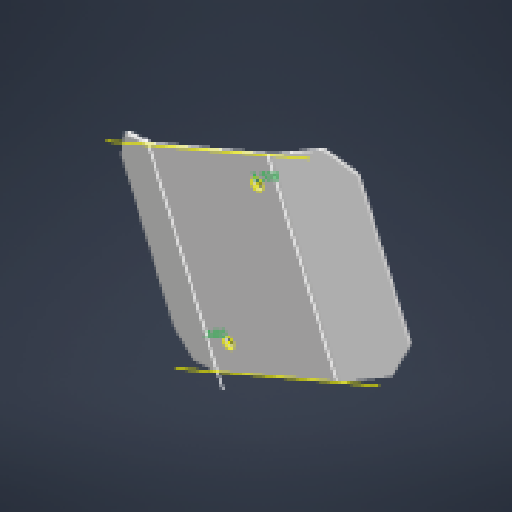
# Autodesk Inventor part: aligner
Saved by Autodesk Inventor 2025.2 (Build 292293000, 293)
## iProperties
Created: 2026-01-05
Part Number: aligner
Material: Acetal Resin, Black
Document SubType Name: Modeling
Designer: cloudy
Density: 1.425 g/cm^3
Appearance: Smooth - Black
Author: cloudy
Autodesk Inventor part; units mm, degrees
ref_plane "YZ Plane" through (0, 0, 0) normal (1, 0, 0) x (0, 1, 0)
ref_plane "XZ Plane" through (0, 0, 0) normal (0, 1, 0) x (-1, 0, 0)
ref_plane "XY Plane" through (0, 0, 0) normal (0, 0, 1) x (1, 0, 0)
sketch "Sketch1" plane through (0, 0, 0) normal (0, 0, 1) x (1, 0, 0)
  circle A0 centre (0, 0) radius 3.0353 construction
  circle A1 centre (16.5589, 87.3442) radius 3.0353 construction
  line L0 (98.2753, 26.7063) -> (-41.995, -32.8756)
  line L1 (-41.995, -32.8756) -> (-81.7163, 60.6379)
  line L2 (-81.7163, 60.6379) -> (58.554, 120.2198)
  line L3 (58.554, 120.2198) -> (98.2753, 26.7063)
  line L4 (98.2753, 26.7063) -> (-81.7163, 60.6379) construction
  line L5 (-41.995, -32.8756) -> (58.554, 120.2198) construction
  line L6 (28.1401, -3.0847) -> (-11.5812, 90.4289) construction
  line L7 (-55.6349, 168.7379) -> (0.8706, 192.7395) projected
  circle A2 centre (16.5589, 87.3442) radius 2.1844
  circle A3 centre (0, 0) radius 2.1844
  point P0 (0, 0)
  point P1 (8.2795, 43.6721)
  dimension "d0" = 101.6
  dimension "d1" = 152.4
  dimension "d5" = 49.3889
  dimension "d6" = 49.3889
  dimension "d7" = 13.8407
  dimension "d8" = 13.8407
  dimension "d22" = 4.3688
  dimension "d23" = 4.3688
  constraints: 14 end point, 4 midpoint, 3 parallel, 2 centre point, 2 coincident, 1 perpendicular
  measures "d0" distance of L0.end L1.end
  measures "d1" distance of L1.end L2.end
  measures "d5" diameter of A0.centre L6
  measures "d6" diameter of A1.centre L6
  measures "d7" distance from line of L2 A1.centre
  measures "d8" distance from line of L0 A0.centre
  measures "d22" diameter of A2
  measures "d23" diameter of A3
extrude "Extrusion1" add sketch "Sketch1" along normal blind 2.54
chamfer "Chamfer1" distance 12.7 angle 45 4 edges at (98.2753, 26.7063, 1.27) (58.554, 120.2198, 1.27) (-81.7163, 60.6379, 1.27) (-41.995, -32.8756, 1.27)
sketch "Sketch2" plane through (0, 0, 2.54) normal (0, 0, 1) x (1, 0, 0)
  line L0 (-30.3058, -27.9105) -> (86.5861, 21.7412) projected
  line L1 (62.5583, 11.535) -> (22.837, 105.0485)
  line L2 (46.8648, 115.2547) -> (-70.0271, 65.603) projected
  line L3 (-47.1373, 78.4883) -> (-3.2385, -24.8602)
  circle A0 centre (16.5589, 87.3442) radius 2.1844 projected
  point P0 (0, 0)
  point P1 (0, 0)
  dimension "d14" = 12.7
  dimension "d24" = 12.7
  constraints: 4 end point, 2 perpendicular, 2 point on line
  measures "d14" distance from line of L3 point (0, 0)
  measures "d24" distance from line of L1 A0.centre
bend part "Bend Part1" radius 6.35 angle 20 line through (62.5583, 11.535, 2.54) along (-0.3909577, 0.9204086, 0) centre toward (0, 0, -1) moving side (0.9204086, 0.3909577, 0) both sides no
bend part "Bend Part2" radius 6.35 angle 20 line through (-47.1373, 78.4883, 2.54) along (0.3909577, -0.9204086, 0) centre toward (0, 0, -1) moving side (-0.9204086, -0.3909577, 0) both sides no
equation "\"d5\" = d6"
equation "\"d7\" = d8"
body "Solid1"
